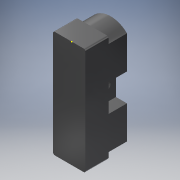
# Autodesk Inventor part: sensor
Saved by Autodesk Inventor 2017 (Build 210142000, 142)
## iProperties
Created: 2015-04-04
Part Number: sensor
Material: Rubber
Document SubType Name: Modeling
Designer: George
Density: 0.93 g/cm^3
Appearance: Rubber - Black - Version 1.1
Author: George
Autodesk Inventor part; units mm, degrees
ref_plane "YZ Plane" through (0, 0, 0) normal (1, 0, 0) x (0, 1, 0)
sketch "Sketch1" plane through (0, 0, 0) normal (0, 1, 0) x (-1, 0, 0)
  line L0 (0, 0) -> (17.6, 0)
  line L1 (17.6, 0) -> (17.6, -58)
  line L2 (17.6, -58) -> (0, -58)
  line L3 (0, -58) -> (0, 0)
  dimension "d0" = 58
  dimension "d1" = 17.6
  constraints: 8 end point, 2 parallel, 1 horizontal, 1 perpendicular
  measures "d0" distance of L0.end L1.end
  measures "d1" distance of L0.start L0.end
extrude "Extrusion1" add sketch "Sketch1" along normal blind 22.5
ref_plane "Work Plane1" through (0, 0, -29) normal (0, 0, -1) x (-1, 0, 0)
fillet "Fillet1" radius 1 1 edges at (-17.6, 11.25, -58)
mirror "Mirror1" about plane through (0, 0, -29) normal (0, 0, -1) of "Fillet1"
ref_plane "Work Plane2" through (-8.8, 0, -57) normal (-1, 0, 0) x (0, 0, 1)
mirror "Mirror2" about plane through (-8.8, 0, -57) normal (-1, 0, 0) of "Fillet1", "Mirror1"
sketch "Sketch2" plane through (0, 22.5, 0) normal (0, 1, 0) x (1, 0, 0)
  line L0 (-17.6, 57) -> (-17.6, 1) projected
  line L1 (-17.6, 21.5) -> (-7.5, 21.5)
  line L2 (-7.5, 21.5) -> (-7.5, 36.5)
  line L3 (-7.5, 36.5) -> (-17.6, 36.5)
  line L4 (-17.6, 36.5) -> (-17.6, 21.5)
  line L5 (0, 1) -> (0, 57) projected
  line L6 (-16.6, 0) -> (-1, 0) projected
  line L7 (0, 57) -> (0, 1) projected
  line L8 (0, 21.5) -> (-6, 21.5)
  line L9 (-6, 21.5) -> (-6, 36.5)
  line L10 (-6, 36.5) -> (0, 36.5)
  line L11 (0, 36.5) -> (0, 21.5)
  point P0 (0, 0)
  dimension "d5" = 15
  dimension "d6" = 10.1
  dimension "d7" = 21.5
  dimension "d10" = 1.5
  constraints: 16 end point, 4 parallel, 2 horizontal, 2 perpendicular, 2 point on line
  measures "d5" distance of L1.end L2.end
  measures "d6" distance of L2.end L3.end
  measures "d7" distance between parallel lines of L6 L1
  measures "d10" distance between parallel lines of L9 L2
extrude "Extrusion3" cut sketch "Sketch2" against normal blind 10
sketch "Sketch3" plane through (-7.5, 22.5, -36.5) normal (-1, 0, 0) x (0, 0, 1)
  point P0 (36.5, -22.5)
sketch "Sketch4" plane through (-7.5, 22.5, -36.5) normal (-1, 0, 0) x (0, 0, 1)
  circle A0 centre (7.5, -5) radius 2.1
  line L0 (0, 0) -> (15, 0) projected
  line L1 (0, 0) -> (0, -10) projected
  point P0 (36.5, -22.5)
  dimension "d13" = 4.2
  dimension "d14" = 5
  dimension "d15" = 7.5
  constraints: 1 centre point
  measures "d13" diameter of A0
  measures "d14" distance from line of L0 A0.centre
  measures "d15" distance from line of A0.centre L1
extrude "Extrusion4" cut sketch "Sketch4" against normal blind 1.5
sketch "Sketch9" plane through (0, 22.5, 0) normal (0, 1, 0) x (1, 0, 0)
  arc A0 (-17.6, 3.6225) -> (-8.8, 0) centre (-8.8, 12.5) ccw
  line L0 (-16.6, 0) -> (-1, 0) projected
  line L1 (-17.6, 21.5) -> (-17.6, 1) projected
  line L2 (-1, 0) -> (-16.6, 0) projected
  line L3 (-8.8, 0) -> (-17.6, 0)
  line L4 (-17.6, 0) -> (-17.6, 3.6225)
  point P0 (0, 0)
  dimension "d20" = 25
  dimension "d21" = 8.8
  constraints: 4 end point, 2 point on circle, 2 tangent, 1 centre point, 1 midpoint, 1 perpendicular, 1 point on line
  measures "d20" diameter of A0
  measures "d21" distance from line of L1 A0.centre
extrude "Extrusion5" cut sketch "Sketch9" against normal blind 10
mirror "Mirror3" about plane through (0, 0, -29) normal (0, 0, -1) of "Extrusion5"
mirror "Mirror4" about plane through (-8.8, 0, -57) normal (-1, 0, 0) of "Extrusion5", "Mirror3"
shell "Shell1" thickness 1 removed faces 1 at (-14.2333, 22.5, -42.4592)
body "Solid1"
